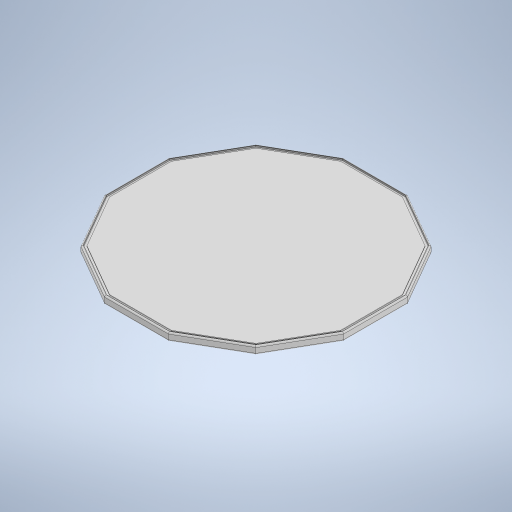
# Autodesk Inventor part: (x2)_POSPA_Large_Bottom
Saved by Autodesk Inventor 2024 (Build 280153000, 153)
## iProperties
Created: 2023-12-08
Part Number: (x2)_POSPA_Large_Bottom
Material: 일반
Document SubType Name: Modeling
Designer: jsw
Density: 1 g/cm^3
Appearance: 기본값
Author: jsw
Autodesk Inventor part; units mm, degrees
ref_plane "YZ Plane" through (0, 0, 0) normal (1, 0, 0) x (0, 1, 0)
ref_plane "XZ Plane" through (0, 0, 0) normal (0, 1, 0) x (-1, 0, 0)
ref_plane "XY Plane" through (0, 0, 0) normal (0, 0, 1) x (1, 0, 0)
sketch "스케치1" plane through (0, 0, 0) normal (0, 1, 0) x (-1, 0, 0)
  line L0 (-74.8338, 74.8338) -> (-27.3911, 102.2249)
  line L1 (-27.3911, 102.2249) -> (27.3911, 102.2249)
  line L2 (27.3911, 102.2249) -> (74.8338, 74.8338)
  line L3 (74.8338, 74.8338) -> (102.2249, 27.3911)
  line L4 (102.2249, 27.3911) -> (102.2249, -27.3911)
  line L5 (102.2249, -27.3911) -> (74.8338, -74.8338)
  line L6 (74.8338, -74.8338) -> (27.3911, -102.2249)
  line L7 (27.3911, -102.2249) -> (-27.3911, -102.2249)
  line L8 (-27.3911, -102.2249) -> (-74.8338, -74.8338)
  line L9 (-74.8338, -74.8338) -> (-102.2249, -27.3911)
  line L10 (-102.2249, -27.3911) -> (-102.2249, 27.3911)
  line L11 (-102.2249, 27.3911) -> (-74.8338, 74.8338)
  line L12 (105.4249, -28.2485) -> (77.1764, -77.1764)
  line L13 (77.1764, -77.1764) -> (28.2485, -105.4249)
  line L14 (28.2485, -105.4249) -> (-28.2485, -105.4249)
  line L15 (-28.2485, -105.4249) -> (-77.1764, -77.1764)
  line L16 (-77.1764, -77.1764) -> (-105.4249, -28.2485)
  line L17 (-105.4249, -28.2485) -> (-105.4249, 28.2485)
  line L18 (-105.4249, 28.2485) -> (-77.1764, 77.1764)
  line L19 (-77.1764, 77.1764) -> (-28.2485, 105.4249)
  line L20 (-28.2485, 105.4249) -> (28.2485, 105.4249)
  line L21 (28.2485, 105.4249) -> (77.1764, 77.1764)
  line L22 (77.1764, 77.1764) -> (105.4249, 28.2485)
  line L23 (105.4249, 28.2485) -> (105.4249, -28.2485)
  point P0 (0, 0)
  point P1 (0, 0)
  point P2 (0, 0)
  dimension "d0" = 211.662
  dimension "d1" = 3.2
  constraints: 48 end point, 2 coincident, 2 horizontal, 50 other
  measures "d0" distance of L8.end L2.end
  measures "d1" distance between parallel lines of L3 L22
extrude "돌출1" add sketch "스케치1" along normal blind 6.8 contours L0 L1 L2 L3 L4 L5 L6 L7 L8 L9 L10 L11 | L12 L13 L14 L15 L16 L17 L18 L19 L20 L21 L22 L23
sketch "스케치2" plane through (0, 6.8, 0) normal (0, 1, 0) x (1, 0, 0)
  line L0 (-27.8198, 103.8249) -> (27.8198, 103.8249)
  line L1 (27.8198, 103.8249) -> (76.0051, 76.0051)
  line L2 (76.0051, 76.0051) -> (103.8249, 27.8198)
  line L3 (103.8249, 27.8198) -> (103.8249, -27.8198)
  line L4 (103.8249, -27.8198) -> (76.0051, -76.0051)
  line L5 (76.0051, -76.0051) -> (27.8198, -103.8249)
  line L6 (27.8198, -103.8249) -> (-27.8198, -103.8249)
  line L7 (-27.8198, -103.8249) -> (-76.0051, -76.0051)
  line L8 (-76.0051, -76.0051) -> (-103.8249, -27.8198)
  line L9 (-103.8249, -27.8198) -> (-103.8249, 27.8198)
  line L10 (-103.8249, 27.8198) -> (-76.0051, 76.0051)
  line L11 (-76.0051, 76.0051) -> (-27.8198, 103.8249)
  line L12 (-105.4249, 28.2485) -> (-105.4249, -28.2485) projected
  line L13 (27.2839, -101.8249) -> (-27.2839, -101.8249)
  line L14 (-27.2839, -101.8249) -> (-74.541, -74.541)
  line L15 (-74.541, -74.541) -> (-101.8249, -27.2839)
  line L16 (-101.8249, -27.2839) -> (-101.8249, 27.2839)
  line L17 (-101.8249, 27.2839) -> (-74.541, 74.541)
  line L18 (-74.541, 74.541) -> (-27.2839, 101.8249)
  line L19 (-27.2839, 101.8249) -> (27.2839, 101.8249)
  line L20 (27.2839, 101.8249) -> (74.541, 74.541)
  line L21 (74.541, 74.541) -> (101.8249, 27.2839)
  line L22 (101.8249, 27.2839) -> (101.8249, -27.2839)
  line L23 (101.8249, -27.2839) -> (74.541, -74.541)
  line L24 (74.541, -74.541) -> (27.2839, -101.8249)
  point P0 (0, 0)
  point P1 (0, 0)
  point P2 (0, 0)
  dimension "d4" = 1.6
  dimension "d5" = 2
  constraints: 48 end point, 2 coincident, 2 horizontal, 50 other
  measures "d4" distance between parallel lines of L9 L12
  measures "d5" distance between parallel lines of L16 L9
extrude "돌출2" cut sketch "스케치2" against normal blind 1.2
sketch "스케치5" plane through (0, 6.8, 0) normal (0, 1, 0) x (1, 0, 0)
  line L0 (-74.541, -74.541) -> (-27.2839, -101.8249) projected
  line L1 (-27.2839, -101.8249) -> (27.2839, -101.8249) projected
  line L2 (27.2839, -101.8249) -> (74.541, -74.541) projected
  line L3 (74.541, -74.541) -> (101.8249, -27.2839) projected
  line L4 (101.8249, -27.2839) -> (101.8249, 27.2839) projected
  line L5 (101.8249, 27.2839) -> (74.541, 74.541) projected
  line L6 (74.541, 74.541) -> (27.2839, 101.8249) projected
  line L7 (27.2839, 101.8249) -> (-27.2839, 101.8249) projected
  line L8 (-27.2839, 101.8249) -> (-74.541, 74.541) projected
  line L9 (-74.541, 74.541) -> (-101.8249, 27.2839) projected
  line L10 (-101.8249, 27.2839) -> (-101.8249, -27.2839) projected
  line L11 (-101.8249, -27.2839) -> (-74.541, -74.541) projected
  point P0 (0, 0)
extrude "돌출5" cut sketch "스케치5" against normal blind 0.6
fillet "모깎기1" radius 1.2 24 edges at (91.3006, 0, 52.7124) (91.3006, 6.8, 52.7124) (105.4249, 6.8, 0) (105.4249, 0, 0) (91.3006, 6.8, -52.7124) (91.3006, 0, -52.7124) (52.7124, 6.8, -91.3006) (52.7124, 0, -91.3006) (0, 0, -105.4249) (0, 6.8, -105.4249) (-52.7124, 6.8, -91.3006) (-52.7124, 0, -91.3006) (-91.3006, 0, -52.7124) (-91.3006, 6.8, -52.7124) (-105.4249, 0, 0) (-105.4249, 6.8, 0) (-91.3006, 0, 52.7124) (-91.3006, 6.8, 52.7124) (-52.7124, 0, 91.3006) (-52.7124, 6.8, 91.3006) (0, 0, 105.4249) (0, 6.8, 105.4249) (52.7124, 0, 91.3006) (52.7124, 6.8, 91.3006)
sketch "스케치7" plane through (0, 0, 0) normal (0, -1, 0) x (1, 0, 0)
  line L0 (10, -7.5) -> (-10, -7.5)
  line L1 (-10, -7.5) -> (-10, -2.5)
  line L2 (-10, -2.5) -> (10, -2.5)
  line L3 (10, -2.5) -> (10, -7.5)
  line L4 (10, -7.5) -> (-10, -2.5) construction
  line L5 (-10, -7.5) -> (10, -2.5) construction
  line L6 (0, 0) -> (-24.3026, 0)
  line L7 (10, 7.5) -> (-10, 7.5)
  line L8 (-10, 7.5) -> (-10, 2.5)
  line L9 (-10, 2.5) -> (10, 2.5)
  line L10 (10, 2.5) -> (10, 7.5)
  line L11 (10, 7.5) -> (-10, 2.5) construction
  line L12 (-10, 7.5) -> (10, 2.5) construction
  point P0 (0, -5)
  point P1 (0, 5)
  dimension "d26" = 20
  dimension "d27" = 5
  dimension "d28" = 2.5
  constraints: 26 end point, 5 symmetric about line, 2 horizontal, 2 midpoint, 2 parallel, 1 perpendicular, 1 vertical alignment
  measures "d26" distance of L0.start L0.end
  measures "d27" distance of L0.end L1.end
  measures "d28" distance from line of L2 L6.start
extrude "돌출7" add sketch "스케치7" along normal blind 10
sketch "스케치8" plane through (-10, 0, 7.5) normal (0, 0, 1) x (1, 0, 0)
  circle A0 centre (15, -5) radius 1.25
  line L0 (-17.927, 0) -> (37.927, 0) projected
  line L1 (20, 0) -> (20, -10) projected
  line L2 (20, -10) -> (0, -10) projected
  line L3 (10, -10) -> (10, 0)
  circle A1 centre (5, -5) radius 1.25
  point P0 (20, -5)
  dimension "d31" = 2.5
  dimension "d32" = 5
  dimension "d33" = 5
  constraints: 2 centre point, 2 end point, 2 midpoint, 1 perpendicular, 1 symmetric about line, 1 other
  measures "d31" diameter of A0
  measures "d32" distance from line of A0.centre L0
  measures "d33" distance of point (20, -5) A0.centre
extrude "돌출8" cut sketch "스케치8" against normal up to surface (15 mm away) contours A0 | A1
